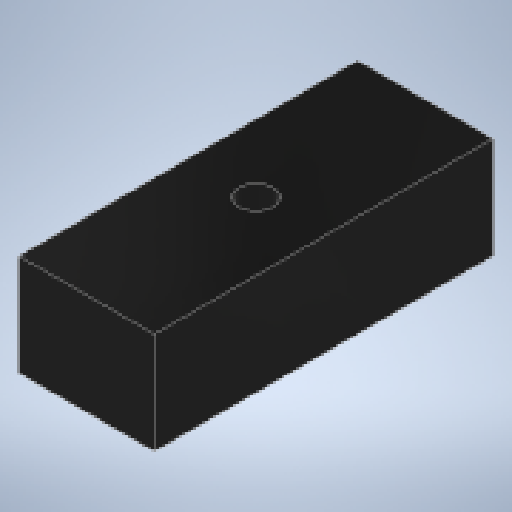
# Autodesk Inventor part: Base_Plate_Spacer
Saved by Autodesk Inventor 2025.1 (Build 291241020, 241B)
## iProperties
Created: 2024-11-14
Part Number: Base_Plate_Spacer
Material: PC/ABS Plastic
Document SubType Name: Modeling
Designer: leon-
Density: 1.1 g/cm^3
Appearance: Smooth - Black
Author: leon-
Autodesk Inventor part; units mm, degrees
ref_plane "YZ Plane" through (0, 0, 0) normal (1, 0, 0) x (0, 1, 0)
ref_plane "XZ Plane" through (0, 0, 0) normal (0, 1, 0) x (-1, 0, 0)
ref_plane "XY Plane" through (0, 0, 0) normal (0, 0, 1) x (1, 0, 0)
sketch "Sketch1" plane through (0, 0, 0) normal (0, 1, 0) x (-1, 0, 0)
  line L0 (0, 0) -> (20, 0)
  line L1 (20, 0) -> (20, -50)
  line L2 (20, -50) -> (0, -50)
  line L3 (0, -50) -> (0, 0)
  dimension "d0" = 50
  dimension "d1" = 20
  constraints: 8 end point, 2 parallel, 1 horizontal, 1 perpendicular
  measures "d0" distance of L0.end L1.end
  measures "d1" distance of L1.end L2.end
extrude "Extrusion1" add sketch "Sketch1" along normal blind 15
sketch "Sketch2" plane through (0, 15, 0) normal (0, 1, 0) x (1, 0, 0)
  line L0 (-20, 50) -> (-20, 0) projected
  line L1 (0, 50) -> (-20, 50) projected
  point P0 (0, 0)
  point P1 (-10, 25)
  point P2 (-20, 25)
  point P3 (-10, 50)
  dimension "d5" = 10
  dimension "d6" = 25
  constraints: 2 midpoint
  measures "d5" distance from line of L0 point (-10, 25)
  measures "d6" distance of point (-10, 50) point (-10, 25)
hole "Hole1" at (-10, 15, -25) direction (0, -1, 0) diameter 5 end through all
body "Solid1"
